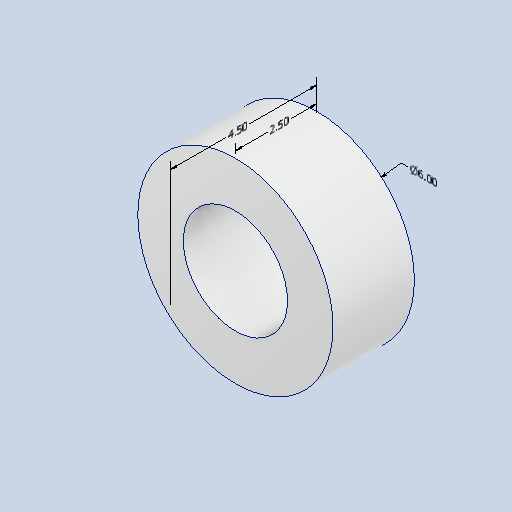
# Autodesk Inventor part: bearing_3_6_2.5_noscrew
Saved by Autodesk Inventor 2024.1 (Build 281209000, 209)
## iProperties
Created: 2024-11-28
Part Number: bearing_3_6_2.5_noscrew
Material: アルミニウム 6061
Document SubType Name: Modeling
Designer: hibik
Density: 2.7 g/cm^3
Appearance: アルミニウム - フラット
Author: hibik
Autodesk Inventor part; units mm, degrees
ref_plane "YZ Plane" through (0, 0, 0) normal (1, 0, 0) x (0, 1, 0)
ref_plane "XZ Plane" through (0, 0, 0) normal (0, 1, 0) x (-1, 0, 0)
sketch "スケッチ1" plane through (0, 0, 0) normal (0, 0, 1) x (1, 0, 0)
  circle A0 centre (0, 0) radius 1.6
  circle A1 centre (0, 0) radius 3
  dimension "d0" = 3.2
  dimension "d1" = 6
  constraints: 2 centre point, 2 coincident
  measures "d0" diameter of A0
  measures "d1" diameter of A1
extrude "押し出し1" add sketch "スケッチ1" along normal blind 2.5
sketch "スケッチ2" plane through (0, 0, 0) normal (1, 0, 0) x (0, 1, 0)
  arc A0 (2.85, 3.5) -> (-2.85, 3.5) centre (0, -0.0613) ccw
  line L0 (2.85, 3.5) -> (-2.85, 3.5)
  line L1 (-2.85, 3.5) -> (-2.85, 2.5)
  line L2 (-2.85, 2.5) -> (2.85, 2.5)
  line L3 (2.85, 2.5) -> (2.85, 3.5)
  line L4 (3, 2.5) -> (-3, 2.5) projected
  line L5 (10, 4.5) -> (-10, 4.5)
  line L6 (0, 2.5) -> (0, 4.5)
  point P0 (0, 0)
  point P1 (0, 4.5)
  dimension "d4" = 1
  dimension "d5" = 1
  dimension "d7" = 5.7
  constraints: 12 end point, 3 midpoint, 2 horizontal, 2 parallel, 2 point on circle, 2 vertical alignment, 1 centre point, 1 collinear, 1 perpendicular, 1 tangent, 1 vertical
  measures "d4" distance of L2.end L0.start
  measures "d5" distance between parallel lines of L0 L5
  measures "d7" distance of L0.start L0.end
revolve "回転1" add sketch "スケッチ2" angle 360 about axis through (0, 0, 2.5) along (0, 0, 1) picked at (1.6112, 3.682) contours L0 L6 A0 | L3 L2 L6 L0
ref_plane "作業平面1" through (0, 0, 4.5) normal (0, 0, 1) x (1, 0, 0)
sketch "スケッチ3" plane through (0, 0, 4.5) normal (0, 0, 1) x (1, 0, 0)
  line L0 (2.25, -0.5) -> (-2.25, -0.5)
  line L1 (-2.25, -0.5) -> (-2.25, 0.5)
  line L2 (-2.25, 0.5) -> (2.25, 0.5)
  line L3 (2.25, 0.5) -> (2.25, -0.5)
  line L4 (2.25, -0.5) -> (-2.25, 0.5) construction
  line L5 (-2.25, -0.5) -> (2.25, 0.5) construction
  line L6 (-0.5, -2.25) -> (0.5, -2.25)
  line L7 (0.5, -2.25) -> (0.5, 2.25)
  line L8 (0.5, 2.25) -> (-0.5, 2.25)
  line L9 (-0.5, 2.25) -> (-0.5, -2.25)
  line L10 (-0.5, -2.25) -> (0.5, 2.25) construction
  line L11 (0.5, -2.25) -> (-0.5, 2.25) construction
  point P0 (0, 0)
  point P1 (-0.5, 0.5)
  point P2 (-0.5, -0.5)
  point P3 (0.5, -0.5)
  point P4 (0.5, 0.5)
  dimension "d9" = 4.5
  dimension "d10" = 1
  constraints: 24 end point, 4 midpoint, 4 parallel, 4 perpendicular, 2 horizontal
  measures "d9" distance of L1.end L2.end
  measures "d10" distance of L0.end L1.end
extrude "押し出し2" cut sketch "スケッチ3" against normal blind 1
sketch "スケッチ5" plane through (0, 0, 2.5) normal (0, 0, 1) x (1, 0, 0)
  circle A0 centre (0, 0) radius 3 projected
extrude "押し出し4" cut sketch "スケッチ5" along normal through all
